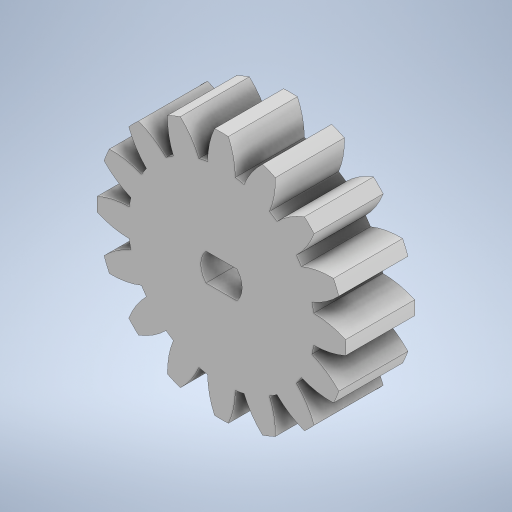
# Autodesk Inventor part: 피니언
Saved by Autodesk Inventor 2024 (Build 280153000, 153)
## iProperties
Created: 2023-09-21
Part Number: 피니언
Material: 일반
Document SubType Name: Modeling
Designer: user
Density: 1 g/cm^3
Appearance: 기본값
Author: user
Autodesk Inventor part; units mm, degrees
ref_plane "YZ Plane" through (0, 0, 0) normal (1, 0, 0) x (0, 1, 0)
ref_plane "XZ Plane" through (0, 0, 0) normal (0, 1, 0) x (-1, 0, 0)
ref_plane "XY Plane" through (0, 0, 0) normal (0, 0, 1) x (1, 0, 0)
sketch "스케치1" plane through (0, 0, 0) normal (0, 0, 1) x (1, 0, 0)
  circle A0 centre (0, 0) radius 18
  dimension "d0" = 36
  constraints: 1 centre point, 1 coincident
  measures "d0" diameter of A0
extrude "돌출1" add sketch "스케치1" along normal mid plane 10
sketch "스케치2" plane through (0, 0, 5) normal (0, 0, 1) x (1, 0, 0)
  circle A0 centre (0, 0) radius 18 projected
  circle A1 centre (0, 0) radius 13.5
  line L0 (0, 0) -> (0, 22.2867) construction
  line L1 (-1, 0) -> (-1, 22.2867) construction
  line L2 (-2, 0) -> (-2, 22.2867) construction
  arc A2 (-1, 17.9722) -> (-2, 13.351) centre (9.3, 13.3246) ccw
  arc A3 (2, 13.351) -> (1, 17.9722) centre (-9.3, 13.3246) ccw
  point P0 (1, 17.9722)
  point P1 (2, 13.351)
  dimension "d3" = 4.5
  dimension "d4" = 1
  dimension "d5" = 1
  dimension "d6" = 11.3
  constraints: 6 end point, 4 point on circle, 3 symmetric about line, 2 centre point, 2 parallel, 2 point on line, 1 vertical, 6 other
  measures "d4" distance between parallel lines of L0 L1
  measures "d5" distance between parallel lines of L1 L2
  measures "d6" radius of A2
extrude "돌출2" cut sketch "스케치2" against normal blind 15 contours A0 A2 A1 A3 picked at (16.1915, -2.5264)
pattern_circular "원형 패턴1" count 16 over 360 about axis through (0, 0, 5) along (0, 0, -1)
sketch "스케치3" plane through (0, 0, 5) normal (0, 0, 1) x (1, 0, 0)
  arc A0 (2, 13.351) -> (1, 17.9722) centre (-9.3, 13.3246) ccw projected
  arc A1 (1, 17.9722) -> (-1, 17.9722) centre (0, 0) ccw projected
  arc A2 (-1, 17.9722) -> (-2, 13.351) centre (9.3, 13.3246) ccw projected
  arc A3 (-2, 13.351) -> (-3.2615, 13.1001) centre (0, 0) ccw projected
  arc A4 (-3.2615, 13.1001) -> (-5.9538, 16.9868) centre (-13.6911, 8.7513) ccw projected
  arc A5 (-5.9538, 16.9868) -> (-7.8015, 16.2215) centre (0, 0) ccw projected
  arc A6 (-7.8015, 16.2215) -> (-6.957, 11.5694) centre (3.493, 15.8692) ccw projected
  arc A7 (-6.957, 11.5694) -> (-8.0264, 10.8548) centre (0, 0) ccw projected
  arc A8 (-8.0264, 10.8548) -> (-12.0012, 13.4154) centre (-15.998, 2.8458) ccw projected
  arc A9 (-12.0012, 13.4154) -> (-13.4154, 12.0012) centre (0, 0) ccw projected
  arc A10 (-13.4154, 12.0012) -> (-10.8548, 8.0264) centre (-2.8458, 15.998) ccw projected
  arc A11 (-10.8548, 8.0264) -> (-11.5694, 6.957) centre (0, 0) ccw projected
  arc A12 (-11.5694, 6.957) -> (-16.2215, 7.8015) centre (-15.8692, -3.493) ccw projected
  arc A13 (-16.2215, 7.8015) -> (-16.9868, 5.9538) centre (0, 0) ccw projected
  arc A14 (-16.9868, 5.9538) -> (-13.1001, 3.2615) centre (-8.7513, 13.6911) ccw projected
  arc A15 (-13.1001, 3.2615) -> (-13.351, 2) centre (0, 0) ccw projected
  arc A16 (-13.351, 2) -> (-17.9722, 1) centre (-13.3246, -9.3) ccw projected
  arc A17 (-17.9722, 1) -> (-17.9722, -1) centre (0, 0) ccw projected
  arc A18 (-17.9722, -1) -> (-13.351, -2) centre (-13.3246, 9.3) ccw projected
  arc A19 (-13.351, -2) -> (-13.1001, -3.2615) centre (0, 0) ccw projected
  arc A20 (-13.1001, -3.2615) -> (-16.9868, -5.9538) centre (-8.7513, -13.6911) ccw projected
  arc A21 (-16.9868, -5.9538) -> (-16.2215, -7.8015) centre (0, 0) ccw projected
  arc A22 (-16.2215, -7.8015) -> (-11.5694, -6.957) centre (-15.8692, 3.493) ccw projected
  arc A23 (-11.5694, -6.957) -> (-10.8548, -8.0264) centre (0, 0) ccw projected
  arc A24 (-10.8548, -8.0264) -> (-13.4154, -12.0012) centre (-2.8458, -15.998) ccw projected
  arc A25 (-13.4154, -12.0012) -> (-12.0012, -13.4154) centre (0, 0) ccw projected
  arc A26 (-12.0012, -13.4154) -> (-8.0264, -10.8548) centre (-15.998, -2.8458) ccw projected
  arc A27 (-8.0264, -10.8548) -> (-6.957, -11.5694) centre (0, 0) ccw projected
  arc A28 (-6.957, -11.5694) -> (-7.8015, -16.2215) centre (3.493, -15.8692) ccw projected
  arc A29 (-7.8015, -16.2215) -> (-5.9538, -16.9868) centre (0, 0) ccw projected
  arc A30 (-5.9538, -16.9868) -> (-3.2615, -13.1001) centre (-13.6911, -8.7513) ccw projected
  arc A31 (-3.2615, -13.1001) -> (-2, -13.351) centre (0, 0) ccw projected
  arc A32 (-2, -13.351) -> (-1, -17.9722) centre (9.3, -13.3246) ccw projected
  arc A33 (-1, -17.9722) -> (1, -17.9722) centre (0, 0) ccw projected
  arc A34 (1, -17.9722) -> (2, -13.351) centre (-9.3, -13.3246) ccw projected
  arc A35 (2, -13.351) -> (3.2615, -13.1001) centre (0, 0) ccw projected
  arc A36 (3.2615, -13.1001) -> (5.9538, -16.9868) centre (13.6911, -8.7513) ccw projected
  arc A37 (5.9538, -16.9868) -> (7.8015, -16.2215) centre (0, 0) ccw projected
  arc A38 (7.8015, -16.2215) -> (6.957, -11.5694) centre (-3.493, -15.8692) ccw projected
  arc A39 (6.957, -11.5694) -> (8.0264, -10.8548) centre (0, 0) ccw projected
  arc A40 (8.0264, -10.8548) -> (12.0012, -13.4154) centre (15.998, -2.8458) ccw projected
  arc A41 (12.0012, -13.4154) -> (13.4154, -12.0012) centre (0, 0) ccw projected
  arc A42 (13.4154, -12.0012) -> (10.8548, -8.0264) centre (2.8458, -15.998) ccw projected
  arc A43 (10.8548, -8.0264) -> (11.5694, -6.957) centre (0, 0) ccw projected
  arc A44 (11.5694, -6.957) -> (16.2215, -7.8015) centre (15.8692, 3.493) ccw projected
  arc A45 (16.2215, -7.8015) -> (16.9868, -5.9538) centre (0, 0) ccw projected
  arc A46 (16.9868, -5.9538) -> (13.1001, -3.2615) centre (8.7513, -13.6911) ccw projected
  arc A47 (13.1001, -3.2615) -> (13.351, -2) centre (0, 0) ccw projected
  arc A48 (13.351, -2) -> (17.9722, -1) centre (13.3246, 9.3) ccw projected
  arc A49 (17.9722, -1) -> (17.9722, 1) centre (0, 0) ccw projected
  arc A50 (17.9722, 1) -> (13.351, 2) centre (13.3246, -9.3) ccw projected
  arc A51 (13.351, 2) -> (13.1001, 3.2615) centre (0, 0) ccw projected
  arc A52 (13.1001, 3.2615) -> (16.9868, 5.9538) centre (8.7513, 13.6911) ccw projected
  arc A53 (16.9868, 5.9538) -> (16.2215, 7.8015) centre (0, 0) ccw projected
  arc A54 (16.2215, 7.8015) -> (11.5694, 6.957) centre (15.8692, -3.493) ccw projected
  arc A55 (11.5694, 6.957) -> (10.8548, 8.0264) centre (0, 0) ccw projected
  arc A56 (10.8548, 8.0264) -> (13.4154, 12.0012) centre (2.8458, 15.998) ccw projected
  arc A57 (13.4154, 12.0012) -> (12.0012, 13.4154) centre (0, 0) ccw projected
  arc A58 (12.0012, 13.4154) -> (8.0264, 10.8548) centre (15.998, 2.8458) ccw projected
  arc A59 (8.0264, 10.8548) -> (6.957, 11.5694) centre (0, 0) ccw projected
  arc A60 (6.957, 11.5694) -> (7.8015, 16.2215) centre (-3.493, 15.8692) ccw projected
  arc A61 (7.8015, 16.2215) -> (5.9538, 16.9868) centre (0, 0) ccw projected
  arc A62 (5.9538, 16.9868) -> (3.2615, 13.1001) centre (13.6911, 8.7513) ccw projected
  arc A63 (3.2615, 13.1001) -> (2, 13.351) centre (0, 0) ccw projected
  line L0 (-4.0823, 0) -> (5.9538, 0) construction
  line L1 (-2.2361, 2) -> (2.2361, 2)
  line L2 (-2.2361, -2) -> (2.2361, -2)
  arc A64 (-2.2361, 2) -> (-2.2361, -2) centre (0, 0) ccw
  arc A65 (2.2361, -2) -> (2.2361, 2) centre (0, 0) ccw
  point P0 (3, 0)
  point P1 (-3, 0)
  dimension "d13" = 2
  dimension "d14" = 2
  dimension "d15" = 6
  constraints: 6 end point, 6 point on circle, 2 centre point, 2 parallel, 1 coincident, 1 horizontal
  measures "d13" distance between parallel lines of L0 L1
  measures "d14" distance between parallel lines of L0 L2
  measures "d15" distance of point (3, 0) point (-3, 0)
extrude "돌출3" cut sketch "스케치3" against normal through all contours L1 A65 L2 A64
